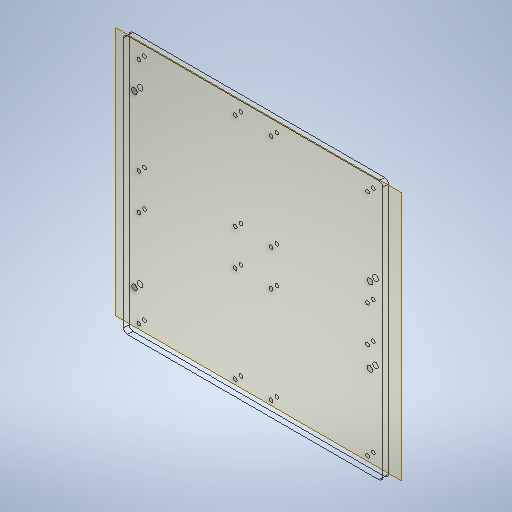
# Autodesk Inventor part: NeoPixel Base
Saved by Autodesk Inventor 2025.1 (Build 291241000, 241)
## iProperties
Created: 2024-11-12
Part Number: NeoPixel Base
Material: Generic
Document SubType Name: Modeling
Designer: benja
Density: 1 g/cm^3
Appearance: Default
Author: benja
Autodesk Inventor part; units mm, degrees
ref_plane "YZ Plane" through (0, 0, 0) normal (1, 0, 0) x (0, 1, 0)
ref_plane "XZ Plane" through (0, 0, 0) normal (0, 1, 0) x (-1, 0, 0)
ref_plane "XY Plane" through (0, 0, 0) normal (0, 0, 1) x (1, 0, 0)
ref_plane "Work Plane1" through (0, 0, 0) normal (0, 0, 1) x (1, 0, 0)
sketch "Sketch1" plane through (0, 0, 0) normal (0, 0, 1) x (1, 0, 0)
  circle A0 centre (61.75, 20) radius 1.5 projected
  circle A1 centre (61.75, -20) radius 1.5 projected
  circle A2 centre (-62.75, 45) radius 1.5 projected
  circle A3 centre (-62.75, -45) radius 1.5 projected
  line L0 (-68.75, 1.5) -> (68.75, 1.5)
  line L1 (68.75, -1.5) -> (-68.75, -1.5)
  line L2 (-68.75, 1.5) -> (68.75, -1.5) construction
  line L3 (68.75, 1.5) -> (-68.75, -1.5) construction
  line L4 (1.5, 60) -> (1.5, -60)
  line L5 (-1.5, -60) -> (-1.5, 60)
  line L6 (-1.5, 60) -> (1.5, -60) construction
  line L7 (1.5, 60) -> (-1.5, -60) construction
  line L8 (-1.5, 1.5) -> (-68.5, 1.5)
  line L9 (-68.5, 1.5) -> (-68.5, 66.5)
  line L10 (-66.5, 68.5) -> (-1.5, 68.5)
  line L11 (-1.5, 68.5) -> (-1.5, 1.5)
  line L12 (-1.5, -1.5) -> (-68.5, -1.5)
  line L13 (-68.5, -1.5) -> (-68.5, -66.5)
  line L14 (-66.5, -68.5) -> (-1.5, -68.5)
  line L15 (-1.5, -68.5) -> (-1.5, -1.5)
  line L16 (1.5, 1.5) -> (68.5, 1.5)
  line L17 (68.5, 1.5) -> (68.5, 68.5)
  line L18 (66.5, 68.5) -> (1.5, 68.5)
  line L19 (1.5, 68.5) -> (1.5, 1.5)
  line L20 (1.5, -1.5) -> (68.5, -1.5)
  line L21 (68.5, -1.5) -> (68.5, -68.5)
  line L22 (66.5, -68.5) -> (1.5, -68.5)
  line L23 (1.5, -68.5) -> (1.5, -1.5)
  circle A4 centre (61.75, -20) radius 1.5
  circle A5 centre (-62.75, 45) radius 1.5
  circle A6 centre (-62.75, -45) radius 1.5
  line L24 (1.5, 1.5) -> (9.5, 1.5)
  line L25 (9.5, 1.5) -> (9.5, 9.5)
  line L26 (9.5, 9.5) -> (1.5, 9.5)
  line L27 (1.5, 9.5) -> (1.5, 1.5)
  line L28 (1.5, 68.5) -> (9.5, 68.5)
  line L29 (9.5, 68.5) -> (9.5, 60.5)
  line L30 (9.5, 60.5) -> (1.5, 60.5)
  line L31 (1.5, 60.5) -> (1.5, 68.5)
  line L32 (68.5, 68.5) -> (60.5, 68.5)
  line L33 (60.5, 68.5) -> (60.5, 60.5)
  line L34 (60.5, 60.5) -> (68.5, 60.5)
  line L35 (68.5, 60.5) -> (68.5, 66.5)
  line L36 (68.5, 1.5) -> (60.5, 1.5)
  line L37 (60.5, 1.5) -> (60.5, 9.5)
  line L38 (60.5, 9.5) -> (68.5, 9.5)
  line L39 (68.5, 9.5) -> (68.5, 1.5)
  line L40 (68.5, -1.5) -> (60.5, -1.5)
  line L41 (60.5, -1.5) -> (60.5, -9.5)
  line L42 (60.5, -9.5) -> (68.5, -9.5)
  line L43 (68.5, -9.5) -> (68.5, -1.5)
  line L44 (68.5, -68.5) -> (60.5, -68.5)
  line L45 (60.5, -68.5) -> (60.5, -60.5)
  line L46 (60.5, -60.5) -> (68.5, -60.5)
  line L47 (68.5, -60.5) -> (68.5, -66.5)
  line L48 (1.5, -68.5) -> (9.5, -68.5)
  line L49 (9.5, -68.5) -> (9.5, -60.5)
  line L50 (9.5, -60.5) -> (1.5, -60.5)
  line L51 (1.5, -60.5) -> (1.5, -68.5)
  line L52 (1.5, -1.5) -> (9.5, -1.5)
  line L53 (9.5, -1.5) -> (9.5, -9.5)
  line L54 (9.5, -9.5) -> (1.5, -9.5)
  line L55 (1.5, -9.5) -> (1.5, -1.5)
  line L56 (-1.5, 68.5) -> (-9.5, 68.5)
  line L57 (-9.5, 68.5) -> (-9.5, 60.5)
  line L58 (-9.5, 60.5) -> (-1.5, 60.5)
  line L59 (-1.5, 60.5) -> (-1.5, 68.5)
  line L60 (-1.5, 1.5) -> (-9.5, 1.5)
  line L61 (-9.5, 1.5) -> (-9.5, 9.5)
  line L62 (-9.5, 9.5) -> (-1.5, 9.5)
  line L63 (-1.5, 9.5) -> (-1.5, 1.5)
  line L64 (-68.5, 68.5) -> (-60.5, 68.5)
  line L65 (-60.5, 68.5) -> (-60.5, 60.5)
  line L66 (-60.5, 60.5) -> (-68.5, 60.5)
  line L67 (-68.5, 60.5) -> (-68.5, 68.5)
  line L68 (-68.5, 1.5) -> (-60.5, 1.5)
  line L69 (-60.5, 1.5) -> (-60.5, 9.5)
  line L70 (-60.5, 9.5) -> (-68.5, 9.5)
  line L71 (-68.5, 9.5) -> (-68.5, 1.5)
  line L72 (-68.5, -1.5) -> (-60.5, -1.5)
  line L73 (-60.5, -1.5) -> (-60.5, -9.5)
  line L74 (-60.5, -9.5) -> (-68.5, -9.5)
  line L75 (-68.5, -9.5) -> (-68.5, -1.5)
  line L76 (-68.5, -68.5) -> (-60.5, -68.5)
  line L77 (-60.5, -68.5) -> (-60.5, -60.5)
  line L78 (-60.5, -60.5) -> (-68.5, -60.5)
  line L79 (-68.5, -60.5) -> (-68.5, -68.5)
  line L80 (-1.7125, -68.5) -> (-9.7125, -68.5)
  line L81 (-1.5, -1.5) -> (-9.5, -1.5)
  line L82 (-9.5, -1.5) -> (-9.5, -9.5)
  line L83 (-9.5, -9.5) -> (-1.5, -9.5)
  line L84 (-1.5, -9.5) -> (-1.5, -1.5)
  circle A7 centre (-9.5, 60.5) radius 1
  circle A8 centre (-9.5, 9.5) radius 1
  circle A9 centre (-60.5, 60.5) radius 1
  circle A10 centre (-60.5, 9.5) radius 1
  circle A11 centre (-60.5, -9.5) radius 1
  circle A12 centre (-60.5, -60.5) radius 1
  circle A13 centre (-9.5, -9.5) radius 1
  circle A14 centre (9.5, -60.5) radius 1
  circle A15 centre (9.5, -9.5) radius 1
  circle A16 centre (9.5, 9.5) radius 1
  circle A17 centre (9.5, 60.5) radius 1
  circle A18 centre (60.5, 60.5) radius 1
  circle A19 centre (60.5, 9.5) radius 1
  circle A20 centre (60.5, -9.5) radius 1
  circle A21 centre (60.5, -60.5) radius 1
  line L85 (-68.5, -1.5) -> (-68.5, 1.5)
  line L86 (68.5, 1.5) -> (68.5, -1.5)
  line L87 (-1.5, 68.5) -> (1.5, 68.5)
  line L88 (-1.5, -68.5) -> (-9.5, -68.5)
  line L89 (-9.5, -68.5) -> (-9.5, -60.5)
  line L90 (-9.5, -60.5) -> (-1.5, -60.5)
  line L91 (-1.5, -60.5) -> (-1.5, -68.5)
  circle A22 centre (-9.5, -60.5) radius 1
  line L92 (-1.5, -68.5) -> (1.5, -68.5)
  arc A23 (66.5, -68.5) -> (68.5, -66.5) centre (66.5, -66.5) ccw
  arc A24 (-68.5, -66.5) -> (-66.5, -68.5) centre (-66.5, -66.5) ccw
  arc A25 (-66.5, 68.5) -> (-68.5, 66.5) centre (-66.5, 66.5) ccw
  arc A26 (68.5, 66.5) -> (66.5, 68.5) centre (66.5, 66.5) ccw
  point P0 (0, 0)
  dimension "d4" = 3
  dimension "d5" = 3
  dimension "d6" = 67
  dimension "d7" = 67
  dimension "d8" = 67
  dimension "d9" = 67
  dimension "d10" = 67
  dimension "d11" = 67
  dimension "d12" = 67
  dimension "d13" = 67
  dimension "d14" = 8
  dimension "d15" = 8
  dimension "d16" = 8
  dimension "d17" = 8
  dimension "d18" = 8
  dimension "d19" = 8
  dimension "d20" = 8
  dimension "d21" = 8
  dimension "d22" = 8
  dimension "d23" = 8
  dimension "d24" = 8
  dimension "d25" = 8
  dimension "d26" = 8
  dimension "d27" = 8
  dimension "d28" = 8
  dimension "d29" = 8
  dimension "d30" = 8
  dimension "d31" = 8
  dimension "d32" = 8
  dimension "d33" = 8
  dimension "d34" = 8
  dimension "d35" = 8
  dimension "d36" = 8
  dimension "d37" = 8
  dimension "d38" = 8
  dimension "d39" = 8
  dimension "d40" = 8
  dimension "d41" = 8
  dimension "d44" = 8
  dimension "d45" = 8
  dimension "d46" = 2
  dimension "d47" = 2
  dimension "d48" = 2
  dimension "d49" = 2
  dimension "d50" = 2
  dimension "d51" = 2
  dimension "d52" = 2
  dimension "d55" = 2
  dimension "d56" = 2
  dimension "d57" = 2
  dimension "d58" = 2
  dimension "d59" = 2
  dimension "d60" = 2
  dimension "d61" = 2
  dimension "d62" = 8
  dimension "d63" = 8
  dimension "d64" = 2
  dimension "d67" = 2
  dimension "d68" = 2
  dimension "d69" = 2
  dimension "d70" = 2
  constraints: 186 end point, 42 parallel, 23 centre point, 22 horizontal, 21 perpendicular, 19 coincident, 17 point on line, 8 point on circle, 8 tangent, 4 midpoint, 3 concentric
  measures "d4" distance of L0.end L1.start
  measures "d5" distance of L4.end L5.start
  measures "d6" distance of L64.start L10.end
  measures "d7" distance of L8.end L64.start
  measures "d8" distance of L14.end L76.start
  measures "d9" distance of L76.start L12.end
  measures "d10" distance of L18.end L17.end
  measures "d11" distance of L17.end L16.end
  measures "d12" distance of L21.end L22.end
  measures "d13" distance of L20.end L21.end
  measures "d14" distance of L26.end L25.end
  measures "d15" distance of L25.end L24.end
  measures "d16" distance of L29.end L30.end
  measures "d17" distance of L28.end L29.end
  measures "d18" distance of L34.end L33.end
  measures "d19" distance of L33.end L32.end
  measures "d20" distance of L37.end L38.end
  measures "d21" distance of L36.end L37.end
  measures "d22" distance of L42.end L41.end
  measures "d23" distance of L41.end L40.end
  measures "d24" distance of L45.end L46.end
  measures "d25" distance of L44.end L45.end
  measures "d26" distance of L50.end L49.end
  measures "d27" distance of L49.end L48.end
  measures "d28" distance of L53.end L54.end
  measures "d29" distance of L52.end L53.end
  measures "d30" distance of L58.end L57.end
  measures "d31" distance of L57.end L56.end
  measures "d32" distance of L61.end L62.end
  measures "d33" distance of L60.end L61.end
  measures "d34" distance of L65.end L66.end
  measures "d35" distance of L64.end L65.end
  measures "d36" distance of L70.end L69.end
  measures "d37" distance of L69.end L68.end
  measures "d38" distance of L73.end L74.end
  measures "d39" distance of L72.end L73.end
  measures "d40" distance of L78.end L77.end
  measures "d41" distance of L77.end L76.end
  measures "d44" distance of L83.end L82.end
  measures "d45" distance of L82.end L81.end
  measures "d46" diameter of A7
  measures "d47" diameter of A8
  measures "d48" diameter of A9
  measures "d49" diameter of A10
  measures "d50" diameter of A11
  measures "d51" diameter of A12
  measures "d52" diameter of A13
  measures "d55" diameter of A15
  measures "d56" diameter of A16
  measures "d57" diameter of A17
  measures "d58" diameter of A18
  measures "d59" diameter of A19
  measures "d60" diameter of A20
  measures "d61" diameter of A21
  measures "d62" distance of L89.end L90.end
  measures "d63" distance of L88.end L89.end
  measures "d64" diameter of A22
  measures "d67" radius of A23
  measures "d68" radius of A24
  measures "d69" radius of A25
  measures "d70" radius of A26
extrude "Extrusion2" add sketch "Sketch1" along normal blind 3 contours L9 L70 A10 L69 L0 | L0 L5 L1 L85 | L69 A10 L70 L9 L66 A9 L65 L10 L57 A7 L58 L11 L5 L62 A8 L61 L0 | L1 L73 A11 L74 L13 | L61 A8 L62 L5 L0 | L9 A25 L10 L65 A9 L66 | L1 L82 A13 L83 L5 L15 L90 A22 L89 L14 L77 A12 L78 L13 L74 A11 L73 | L5 L11 L87 L19 L4 L0 | L0 L4 L1 L5 | L1 L5 L83 A13 L82 | L78 A12 L77 L14 A24 L13 | L4 L26 A16 L25 L0 | L0 L86 L1 L4 | L1 L4 L23 L92 L15 L5 | L25 A16 L26 L4 L19 L30 A17 L29 L18 L33 A18 L34 L17 L38 A19 L37 L0 | L1 L53 A15 L54 L4 | L37 A19 L38 L17 L0 | L1 L41 A20 L42 L21 L46 A21 L45 L22 L49 A14 L50 L23 L4 L54 A15 L53 | L58 A7 L57 L10 L11 | L19 L18 L29 A17 L30 | L1 L21 L42 A20 L41 | L15 L14 L89 A22 L90 | L50 A14 L49 L22 L23 | L34 A18 L33 L18 A26 L17 | L21 A23 L22 L45 A21 L46
body "Solid2"
